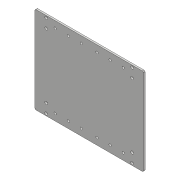
# Autodesk Inventor part: Battery_Base
Saved by Autodesk Inventor 2018 (Build 220112000, 112)
## iProperties
Created: 2019-08-30
Part Number: Battery_Base
Material: Generic
Document SubType Name: Modeling
Designer: Clevo
Density: 1 g/cm^3
Appearance: Default
Author: Clevo
Autodesk Inventor part; units mm, degrees
ref_plane "YZ Plane" through (0, 0, 0) normal (1, 0, 0) x (0, 1, 0)
ref_plane "XZ Plane" through (0, 0, 0) normal (0, 1, 0) x (-1, 0, 0)
ref_plane "XY Plane" through (0, 0, 0) normal (0, 0, 1) x (1, 0, 0)
sketch "Sketch1" plane through (0, 0, 0) normal (0, 1, 0) x (-1, 0, 0)
  line L0 (-78, -83) -> (78, -83)
  line L1 (78, -83) -> (78, 83)
  line L2 (78, 83) -> (-78, 83)
  line L3 (-78, 83) -> (-78, -83)
  line L4 (-78, -83) -> (78, 83) construction
  line L5 (78, -83) -> (-78, 83) construction
  point P0 (0, 0)
  dimension "d0" = 156
  dimension "d1" = 166
  constraints: 12 end point, 2 midpoint, 2 parallel, 1 horizontal, 1 perpendicular
  measures "d0" distance of L1.end L2.end
  measures "d1" distance of L0.end L1.end
extrude "Extrusion1" add sketch "Sketch1" along normal blind 3.175
sketch "Sketch2" plane through (0, 3.175, 0) normal (0, 1, 0) x (1, 0, 0)
  line L0 (64.9, 70.3) -> (14.9, 70.3)
  line L1 (14.9, 70.3) -> (14.9, -70.3)
  line L2 (14.9, -70.3) -> (64.9, -70.3)
  line L3 (64.9, -70.3) -> (64.9, 70.3)
  line L4 (78, 83) -> (-78, 83) projected
  line L5 (78, -83) -> (78, 83) projected
  point P0 (0, 0)
  point P1 (64.9, 0)
  point P2 (39.9, 70.3)
  point P3 (39.9, -70.3)
  dimension "d4" = 50
  dimension "d5" = 12.7
  dimension "d6" = 13.1
  constraints: 8 end point, 3 midpoint, 2 parallel, 1 horizontal, 1 horizontal alignment, 1 perpendicular
  measures "d4" distance of L1.end L2.end
  measures "d5" distance between parallel lines of L4 L0
  measures "d6" distance between parallel lines of L5 L3
hole "Hole1" at (39.9, 3.175, -70.3) at (39.9, 3.175, 70.3) at (64.9, 3.175, -70.3) at (14.9, 3.175, -70.3) at (14.9, 3.175, 70.3) at (64.9, 3.175, 70.3) direction (0, -1, 0) diameter 4.5 end through all clearance for "Flat Head Machine Screw" size "M4" standard "Ansi Metric M Profile"
mirror "Mirror1" about plane through (0, 0, 0) normal (1, 0, 0) of "Hole1"
sketch "Sketch3" plane through (-78, 0, -83) normal (-1, 0, 0) x (0, 0, 1)
  line L0 (0, 0) -> (166, 0) projected
  line L1 (166, 0) -> (166, 3.175) projected
  line L2 (0, 3.175) -> (166, 3.175) projected
  line L3 (0, 0) -> (0, 3.175) projected
  point P0 (83, 0)
extrude "Extrusion2" add sketch "Sketch3" along normal blind 25.4
mirror "Mirror2" about plane through (0, 0, 0) normal (1, 0, 0) of "Extrusion2"
sketch "Sketch4" plane through (0, 3.175, 0) normal (0, 1, 0) x (1, 0, 0)
  line L0 (-81.9624, 79.0312) -> (-81.9624, 61.5687)
  circle A0 centre (-64.9, 70.3) radius 2.25 projected
  line L1 (-103.4, -83) -> (-103.4, 83) projected
  point P0 (0, 0)
  point P1 (-81.9624, 70.3)
  dimension "d16" = 17.4625
  dimension "d17" = 21.4376
  constraints: 2 end point, 1 horizontal alignment, 1 midpoint, 1 vertical
  measures "d16" distance of L0.start L0.end
  measures "d17" distance between parallel lines of L1 L0
hole "Hole2" at (-81.9624, 3.175, -61.5687) at (-81.9624, 3.175, -79.0312) direction (0, -1, 0) diameter 5.3 end through all clearance for "Flat Head Machine Screw" size "M5" standard "Ansi Metric M Profile"
mirror "Mirror3" about plane through (0, 0, 0) normal (0, 0, 1) of "Hole2"
mirror "Mirror4" about plane through (0, 0, 0) normal (1, 0, 0) of "Hole2", "Mirror3"
fillet "Fillet1" radius 2 4 edges at (103.4, 1.5875, -83) (103.4, 1.5875, 83) (-103.4, 1.5875, -83) (-103.4, 1.5875, 83)
ref_plane "Work Plane1" through (0, 0, 0) normal (1, 0, 0) x (0, 1, 0)
body "Solid1"
